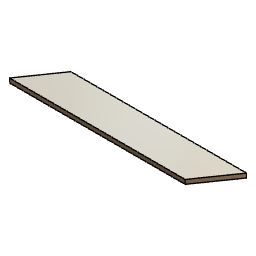
name_sign_bottom_panel (Autodesk Fusion 360 design; units mm, degrees)
Autodesk Fusion 360 part; units mm, degrees
sketch "Name Sign Bottom Panel" plane through (0, 0, 0) normal (1, 0, 0) x (0, 1, 0) in component "Name Sign Bottom Panel"
  line L0 (-0.0158, 146.1836) -> (94.3556, 107.4791)
  line L1 (94.3556, 113.9641) -> (-0.0158, 152.6686)
  line L2 (-0.0158, 152.6686) -> (-0.0158, 146.1836)
  line L3 (94.3556, 113.9641) -> (94.3556, 107.4791)
  dimension "d13" = 102
  dimension "d14" = 6
  dimension "d18" = 67.7
  constraint vertical L2
  constraint parallel L2 L3
  measures "d13" distance of L0.start L0.end
  measures "d14" distance of L0 L1
  measures "d18" angle of L0 L3
extrude "Extrude2" add sketch "Name Sign Bottom Panel" along normal blind 270 in component "Name Sign Bottom Panel"
component "Name Sign Bottom Panel" placed x (1, 0, 0) y (0, 1, 0) z (0, 0, 1) at (0, 0, 0)
equation "MDFThickness = 6 mm" comment "Thickness of the MDF board"
equation "d14 = MDFThickness"
named bodies: "Name Sign Bottom Panel"
